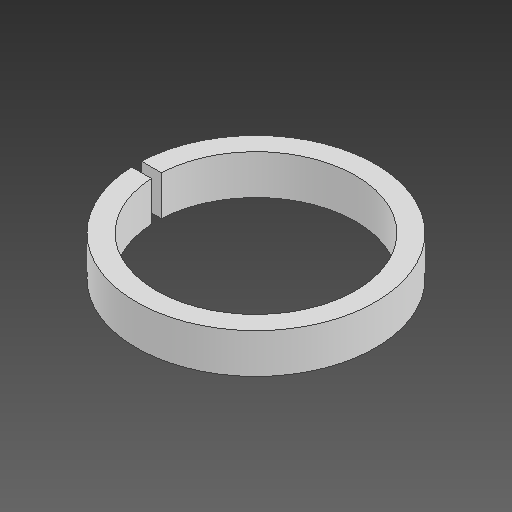
# Autodesk Inventor part: MotorClampUhmw
Saved by Autodesk Inventor 2021 (Build 250183000, 183)
## iProperties
Created: 2021-03-10
Part Number: MotorClampUhmw
Material: Generic
Document SubType Name: Modeling
Designer: tandu
Density: 1 g/cm^3
Appearance: Default
Mass: 17.505 g
Surface Area: 84.3152 cm^2
Volume: 17.505 cm^3
Author: tandu
Autodesk Inventor part; units mm, degrees
ref_plane "YZ Plane" through (0, 0, 0) normal (1, 0, 0) x (0, 1, 0)
ref_plane "XZ Plane" through (0, 0, 0) normal (0, 1, 0) x (-1, 0, 0)
ref_plane "XY Plane" through (0, 0, 0) normal (0, 0, 1) x (1, 0, 0)
sketch "Sketch1" plane through (0, 0, 0) normal (0, 1, 0) x (-1, 0, 0)
  circle A0 centre (0, 0) radius 38.227
  circle A1 centre (0, 0) radius 31.877
  line L0 (-38.227, 1.5875) -> (38.227, 1.5875)
  line L1 (38.227, 1.5875) -> (38.227, -1.5875)
  line L2 (38.227, -1.5875) -> (-38.227, -1.5875)
  line L3 (-38.227, -1.5875) -> (-38.227, 1.5875)
  line L4 (-38.227, 1.5875) -> (38.227, -1.5875) construction
  line L5 (38.227, 1.5875) -> (-38.227, -1.5875) construction
  point P0 (31.8374, 1.5875)
  point P1 (38.194, 1.5875)
  point P2 (38.194, -1.5875)
  point P3 (31.8374, -1.5875)
  dimension "d0" = 76.454
  dimension "d1" = 6.35
  dimension "d4" = 3.175
  constraints: 12 end point, 2 centre point, 2 midpoint, 2 parallel, 1 horizontal, 1 perpendicular
  measures "d0" diameter of A0
  measures "d1" radial gap between concentric circles of A0 A1
  measures "d4" distance of L0.end L1.end
extrude "Extrusion1" add sketch "Sketch1" along normal blind 12.7 contours L0 A1 A0 | A0 L2 A1 | L0 A1 L2 A0 picked at (-33.9907, 0)
body "Solid1"
